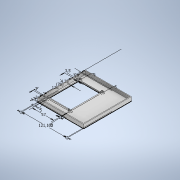
# Autodesk Inventor part: Couvercle supérieur
Saved by Autodesk Inventor 2020 (Build 240168000, 168)
## iProperties
Created: 2020-01-01
Part Number: Couvercle supérieur
Material: Générique
Document SubType Name: Modeling
Designer: Manuel Enzo
Density: 1 g/cm^3
Appearance: Par défaut
Author: Manuel Enzo
Autodesk Inventor part; units mm, degrees
ref_plane "YZ Plane" through (0, 0, 0) normal (1, 0, 0) x (0, 1, 0)
ref_plane "XZ Plane" through (0, 0, 0) normal (0, 1, 0) x (-1, 0, 0)
ref_plane "XY Plane" through (0, 0, 0) normal (0, 0, 1) x (1, 0, 0)
sketch "Esquisse1" plane through (0, 0, 0) normal (0, 1, 0) x (-1, 0, 0)
  line L0 (0, 0) -> (121.1033, 0)
  line L1 (121.1033, 0) -> (121.1033, -126)
  line L2 (121.1033, -126) -> (0, -126)
  line L3 (0, -126) -> (0, 0)
  line L4 (119.1033, -2) -> (2, -2)
  line L5 (2, -2) -> (2, -124)
  line L6 (2, -124) -> (119.1033, -124)
  line L7 (119.1033, -124) -> (119.1033, -2)
  line L8 (114.8533, -24) -> (57.8533, -24)
  line L9 (57.8533, -24) -> (57.8533, -102)
  line L10 (57.8533, -102) -> (114.8533, -102)
  line L11 (114.8533, -102) -> (114.8533, -24)
  circle A0 centre (115.8533, -105.5) radius 2.5
  circle A1 centre (56.8533, -105.5) radius 2.5
  circle A2 centre (56.8533, -21) radius 2.5
  circle A3 centre (115.8533, -21) radius 2.5
  circle A4 centre (56.8533, -21) radius 1
  circle A5 centre (56.8533, -105.5) radius 1
  circle A6 centre (115.8533, -105.5) radius 1
  circle A7 centre (115.8533, -21) radius 1
  dimension "d0" = 126
  dimension "d1" = 121.1033
  dimension "d2" = 2
  dimension "d3" = 2
  dimension "d4" = 2
  dimension "d5" = 2
  dimension "d10" = 4.25
  dimension "d11" = 24
  dimension "d12" = 24
  dimension "d13" = 78
  dimension "d14" = 57
  dimension "d15" = 3
  dimension "d16" = 1
  dimension "d17" = 5
  dimension "d18" = 3
  dimension "d19" = 1
  dimension "d20" = 5
  dimension "d21" = 1
  dimension "d22" = 3.5
  dimension "d23" = 3.5
  dimension "d24" = 1
  dimension "d25" = 5
  dimension "d26" = 5
  dimension "d27" = 1.5
  dimension "d28" = 1.5
  dimension "d29" = 1.5
  dimension "d30" = 1.5
  constraints: 24 end point, 8 centre point, 6 parallel, 4 coincident, 3 horizontal, 3 perpendicular
  measures "d0" distance between parallel lines of L0 L2
  measures "d1" distance between parallel lines of L3 L1
  measures "d2" distance between parallel lines of L2 L6
  measures "d3" distance between parallel lines of L0 L4
  measures "d4" distance between parallel lines of L1 L7
  measures "d5" distance between parallel lines of L3 L5
  measures "d10" distance between parallel lines of L7 L11
  measures "d11" distance between parallel lines of L0 L8
  measures "d12" distance between parallel lines of L2 L10
  measures "d13" distance between parallel lines of L8 L10
  measures "d14" distance between parallel lines of L9 L11
  measures "d15" distance from line of L8 A3.centre
  measures "d16" distance from line of L11 A3.centre
  measures "d17" diameter of A3
  measures "d18" distance from line of L8 A2.centre
  measures "d19" distance from line of L9 A2.centre
  measures "d20" diameter of A2
  measures "d21" distance from line of L11 A0.centre
  measures "d22" distance from line of L10 A0.centre
  measures "d23" distance from line of L10 A1.centre
  measures "d24" distance from line of L9 A1.centre
  measures "d25" diameter of A1
  measures "d26" diameter of A0
  measures "d27" radial gap between concentric circles of A3 A7
  measures "d28" radial gap between concentric circles of A2 A4
  measures "d29" radial gap between concentric circles of A1 A5
  measures "d30" radial gap between concentric circles of A0 A6
extrude "Extrusion1" add sketch "Esquisse1" along normal blind 10 contours L0 L1 L2 L3
extrude "Extrusion2" add sketch "Esquisse1" along normal blind 2 contours L7 L6 L5 L4
extrude "Extrusion3" add sketch "Esquisse1" along normal blind 3 contours A0 | A1 | A2 | A3
